1.3mm_top (Autodesk Fusion 360 design; units mm, degrees)
Autodesk Fusion 360 part; units mm, degrees
sketch "Sketch1" plane through (0, 0, 0) normal (0, 1, 0) x (1, 0, 0)
  line L0 (0, 0) -> (-0.3, 0)
  line L1 (-0.3, 0) -> (-0.3, -0.5895)
  line L2 (-0.3, -0.5895) -> (-0.0332, -0.5895)
  line L3 (0, 0) -> (1.28, 0)
  line L4 (0, -0.46) -> (0, 0)
  line L5 (0.98, -0.46) -> (1.28, -0.38)
  line L6 (1.28, -0.38) -> (1.28, 0)
  line L7 (0, -0.46) -> (0.5, -0.46)
  line L8 (0.5, -0.46) -> (0.5, -0.435)
  line L9 (0.5, -0.435) -> (0.65, -0.435)
  line L10 (0.65, -0.435) -> (0.65, -0.46)
  line L11 (0.65, -0.46) -> (0.98, -0.46)
  line L12 (-0.0075, -0.5571) -> (-0.03, -0.46)
  line L13 (-0.03, -0.46) -> (0, -0.46)
  line L14 (-0.0332, -0.5895) -> (-0.0075, -0.5571)
  line L15 (-0.0332, -0.5895) -> (0, -0.5895) construction
  line L16 (0, -0.5895) -> (-0.0075, -0.5571) construction
  point P0 (0, -0.5895)
  dimension "d2" = 0.5895
  dimension "d7" = 0.3
  dimension "d16" = 1.28
  dimension "d17" = 0.5
  dimension "d18" = 0.15
  dimension "d19" = 0.025
  dimension "d20" = 0.46
  dimension "d29" = 0.08
  dimension "d30" = 0.3
  dimension "d31" = 0.03
  dimension "d32" = 0.0332
  dimension "d33" = 0.0332
  constraint horizontal L0
  constraint vertical L1
  constraint horizontal L2
  constraint coincident L0.start L3.start
  constraint horizontal L3
  constraint vertical L4
  constraint perpendicular L3 L6
  constraint perpendicular L7 L8
  constraint perpendicular L8 L9
  constraint perpendicular L9 L10
  constraint collinear L7 L11
  constraint collinear L7 L13
  constraint coincident P0 L4
  constraint horizontal L11
  constraint coincident P0 L2
  constraint coincident P0 L12
  constraint coincident P0 L15.end
  constraint parallel L2 L15
  measures "d2" distance of L0.end L1.end
  measures "d7" distance of L5.start L6
  measures "d16" distance of L4 L6
  measures "d17" distance of L4.start L7.end
  measures "d18" distance of L8.end L9.end
  measures "d19" distance of L7.end L8.end
  measures "d20" distance of L0.start L7
  measures "d29" distance of L5.end L11
  measures "d30" distance of L1.end P0
  measures "d31" horizontal distance of L4.start L12.end
  measures "d32" distance of P0 L2.end
  measures "d33" distance of P0 L12.start
revolve "Revolve1" add sketch "Sketch1" angle 360 about axis through (0, 0, 0) along (1, 0, 0) makes body 1
sketch "Sketch2" plane through (-0.3, 0, 0) normal (-1, 0, 0) x (0, -1, 0)
  circle A0 centre (0, 0) radius 0.5895
  spline S0 degree 5 poles (-0.5629, -0.1749) (-0.551, -0.1828) (-0.5276, -0.197) (-0.4936, -0.2131) (-0.4507, -0.2248) (-0.4012, -0.2231) (-0.3563, -0.207) (-0.3168, -0.1794) (-0.2846, -0.1471) (-0.2608, -0.1165) (-0.2446, -0.0864) (-0.2356, -0.0538) (-0.2336, -0.0149) (-0.2422, 0.0303) (-0.263, 0.0799) (-0.2918, 0.1324) (-0.3226, 0.1862) (-0.3485, 0.2395) (-0.364, 0.2911) (-0.3667, 0.3397) (-0.3573, 0.3846) (-0.3383, 0.4252) (-0.3129, 0.4611) (-0.2845, 0.4919) (-0.2554, 0.5177) (-0.227, 0.5383) (-0.2054, 0.5507) (-0.1899, 0.5577) (-0.1799, 0.5614) (-0.1749, 0.5629) knots 0 0 0 0 0 0 0.04 0.08 0.12 0.16 0.2 0.24 0.28 0.32 0.36 0.4 0.44 0.48 0.52 0.56 0.6 0.64 0.68 0.72 0.76 0.8 0.84 0.88 0.92 0.96 1 1 1 1 1 1
  line L0 (-0.3883, -0.2378) -> (-0.2412, -0.1121)
  line L1 (-0.23, -0.1) -> (-0.2421, 0.0692)
  spline S1 degree 5 poles (0.1749, -0.5629) (0.1786, -0.5515) (0.1852, -0.529) (0.1929, -0.4962) (0.199, -0.4541) (0.1994, -0.4048) (0.1926, -0.3589) (0.1786, -0.3175) (0.1577, -0.2818) (0.1303, -0.2537) (0.0967, -0.2354) (0.0577, -0.2285) (0.0141, -0.2338) (-0.0332, -0.2502) (-0.0833, -0.2746) (-0.1351, -0.3024) (-0.1876, -0.3288) (-0.2396, -0.3492) (-0.2903, -0.3604) (-0.3385, -0.361) (-0.3835, -0.3519) (-0.4245, -0.3349) (-0.461, -0.3123) (-0.4924, -0.2866) (-0.5185, -0.2592) (-0.5392, -0.2312) (-0.5514, -0.2087) (-0.5581, -0.1918) (-0.5615, -0.1806) (-0.5629, -0.1749) knots 0 0 0 0 0 0 0.04 0.08 0.12 0.16 0.2 0.24 0.28 0.32 0.36 0.4 0.44 0.48 0.52 0.56 0.6 0.64 0.68 0.72 0.76 0.8 0.84 0.88 0.92 0.96 1 1 1 1 1 1
  spline S2 degree 5 poles (0.5629, 0.1749) (0.5515, 0.1786) (0.529, 0.1852) (0.4962, 0.1929) (0.4541, 0.199) (0.4048, 0.1994) (0.3589, 0.1926) (0.3175, 0.1786) (0.2818, 0.1577) (0.2537, 0.1303) (0.2354, 0.0967) (0.2285, 0.0577) (0.2338, 0.0141) (0.2502, -0.0332) (0.2746, -0.0833) (0.3024, -0.1351) (0.3288, -0.1876) (0.3492, -0.2396) (0.3604, -0.2903) (0.361, -0.3385) (0.3519, -0.3835) (0.3349, -0.4245) (0.3123, -0.461) (0.2866, -0.4924) (0.2592, -0.5185) (0.2312, -0.5392) (0.2087, -0.5514) (0.1918, -0.5581) (0.1806, -0.5615) (0.1749, -0.5629) knots 0 0 0 0 0 0 0.04 0.08 0.12 0.16 0.2 0.24 0.28 0.32 0.36 0.4 0.44 0.48 0.52 0.56 0.6 0.64 0.68 0.72 0.76 0.8 0.84 0.88 0.92 0.96 1 1 1 1 1 1
  spline S3 degree 5 poles (-0.1749, 0.5629) (-0.1829, 0.5509) (-0.1971, 0.5272) (-0.2129, 0.4926) (-0.2232, 0.4487) (-0.2203, 0.3986) (-0.2046, 0.3542) (-0.1795, 0.3166) (-0.1485, 0.2863) (-0.1149, 0.2631) (-0.0811, 0.2464) (-0.0479, 0.2363) (-0.0148, 0.2334) (0.023, 0.2417) (0.069, 0.2624) (0.1223, 0.2913) (0.1802, 0.3224) (0.2388, 0.3485) (0.2946, 0.3641) (0.3452, 0.3669) (0.3899, 0.3575) (0.4285, 0.3384) (0.4616, 0.3129) (0.4899, 0.2844) (0.514, 0.2553) (0.5343, 0.2269) (0.5475, 0.2053) (0.5559, 0.1898) (0.5607, 0.1799) (0.5629, 0.1749) knots 0 0 0 0 0 0 0.04 0.08 0.12 0.16 0.2 0.24 0.28 0.32 0.36 0.4 0.44 0.48 0.52 0.56 0.6 0.64 0.68 0.72 0.76 0.8 0.84 0.88 0.92 0.96 1 1 1 1 1 1
  line L2 (-0.0999, 0.6759) -> (-0.25, 0.45)
  line L3 (-0.0883, 0.2312) -> (0.0575, 0.2409)
  circle A1 centre (0, 0) radius 0.5895
  point P0 (-0.3148, -0.1749)
  point P1 (-0.2361, -0.0154)
  point P2 (-0.35, 0.25)
  point P3 (-0.3062, 0.467)
  point P4 (0.1749, -0.3148)
  point P5 (0.0154, -0.2361)
  point P6 (-0.25, -0.35)
  point P7 (-0.467, -0.3062)
  point P8 (0.3148, 0.1749)
  point P9 (0.2361, 0.0154)
  point P10 (0.35, -0.25)
  point P11 (0.3062, -0.467)
  point P12 (-0.1749, 0.3148)
  point P13 (-0.0154, 0.2361)
  point P14 (0.25, 0.35)
  point P15 (0.467, 0.3062)
  dimension "d12" = 360
  constraint coincident A0 S0.start
  constraint coincident A0 S0.end
  constraint midpoint P0 L0
  constraint midpoint P1 L1
  constraint midpoint S0.end L2
  constraint midpoint P13 L3
extrude "Extrude1" add sketch "Sketch2" along normal blind 0.7 separate body contours A0 S0 S1 S2 S3 A1 makes body 2
move_body "Move1" bodies 2 1 to x (0, 0, -1) y (0, 1, 0) z (1, 0, 0) at (0, 0, 0)
combine "Combine1" operation add target body 2 tool bodies 1
equation "d2 = ( 1.179 / 2 ) * 1 mm"
equation "d16 = 2.492 mm - 1.212 mm"
equation "d20 = var / 2"
equation "var = 0.920 mm"
equation "d33 = d32"
